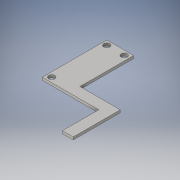
# Autodesk Inventor part: CU1
Saved by Autodesk Inventor 2016 (Build 200138000, 138)
## iProperties
Created: 2018-04-30
Part Number: CU1
Material: Generic
Document SubType Name: Modeling
Designer: Phil Erle
Density: 1 g/cm^3
Appearance: Default
Author: Phil Erle
Autodesk Inventor part; units mm, degrees
ref_plane "YZ Plane" through (0, 0, 0) normal (1, 0, 0) x (0, 1, 0)
ref_plane "XZ Plane" through (0, 0, 0) normal (0, 1, 0) x (-1, 0, 0)
ref_plane "XY Plane" through (0, 0, 0) normal (0, 0, 1) x (1, 0, 0)
sketch "Sketch1" plane through (0, 0, 0) normal (0, 0, 1) x (1, 0, 0)
  line L0 (-10, 40) -> (10, 40)
  line L1 (10, 40) -> (10, 0)
  line L2 (10, 0) -> (40, 0)
  line L3 (40, 0) -> (40, -35)
  line L4 (40, -35) -> (32, -35)
  line L5 (32, -35) -> (32, -8)
  line L6 (32, -8) -> (-10, -8)
  line L7 (-10, -8) -> (-10, 40)
  point P0 (0, 0)
  point P1 (0, 40)
  dimension "d0" = 48
  dimension "d1" = 8
  dimension "d2" = 8
  dimension "d3" = 20
  dimension "d4" = 35
  dimension "d5" = 30
  constraints: 16 end point, 7 perpendicular, 1 horizontal, 1 horizontal alignment, 1 midpoint, 1 vertical alignment
  measures "d0" distance of L6.end L0.start
  measures "d1" distance of L3.end L4.end
  measures "d2" distance between parallel lines of L6 L2
  measures "d3" distance of L0.start L0.end
  measures "d4" distance of L2.end L3.end
  measures "d5" distance of L1.end L2.end
extrude "Extrusion1" add sketch "Sketch1" along normal blind 2
sketch "Sketch2" plane through (0, 0, 2) normal (0, 0, 1) x (1, 0, 0)
  line L0 (-6.5, 36.5) -> (-6.5, -4.5) construction
  line L1 (10, 40) -> (-10, 40) projected
  line L2 (-6.5, 36.5) -> (6.5, 36.5) construction
  point P0 (0, 0)
  point P1 (0, 36.5)
  dimension "d8" = 41
  dimension "d9" = 3.5
  dimension "d17" = 13
  constraints: 4 end point, 3 coincident, 2 vertical alignment, 1 horizontal, 1 midpoint
  measures "d8" distance of L0.start L0.end
  measures "d9" distance from line of L0.start L1
  measures "d17" distance of L2.start L2.end
hole "Hole1" at (-6.5, 36.5, 2) at (-6.5, -4.5, 2) at (6.5, 36.5, 2) direction (0, 0, -1) diameter 4.5 depth 8 tip angle 118 clearance for "Countersunk Flat Head Screw DIN EN ISO 2009" size "M4" standard "DIN"
body "Solid1"
